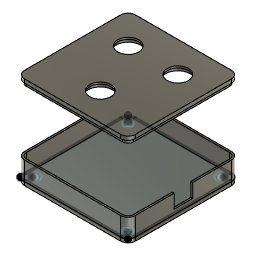
Synthetic_SCG_Actuator_Housing (Autodesk Fusion 360 design; units mm, degrees)
Autodesk Fusion 360 part; units mm, degrees
note: some values were not read from the file. Set by a fixed rule: which sketch regions a step uses.
sketch "Sketch1" plane through (0, 0, 0) normal (0, 0, 1) x (1, 0, 0)
  line L0 (3, 0) -> (55, 0)
  line L1 (58, 3) -> (58, 55)
  line L2 (55, 58) -> (3, 58)
  line L3 (0, 55) -> (0, 3)
  circle A0 centre (4, 54) radius 2.25
  circle A1 centre (54, 54) radius 2.25
  circle A2 centre (54, 4) radius 2.25
  circle A3 centre (4, 4) radius 2.25
  arc A4 (3, 58) -> (0, 55) centre (3, 55) ccw
  arc A5 (58, 55) -> (55, 58) centre (55, 55) ccw
  arc A6 (55, 0) -> (58, 3) centre (55, 3) ccw
  arc A7 (0, 3) -> (3, 0) centre (3, 3) ccw
  line L4 (55, 59) -> (3, 59)
  arc A8 (3, 59) -> (-1, 55) centre (3, 55) ccw
  line L5 (-1, 55) -> (-1, 3)
  arc A9 (-1, 3) -> (3, -1) centre (3, 3) ccw
  line L6 (3, -1) -> (55, -1)
  arc A10 (55, -1) -> (59, 3) centre (55, 3) ccw
  line L7 (59, 3) -> (59, 55)
  arc A11 (59, 55) -> (55, 59) centre (55, 55) ccw
  point P0 (58, 0)
  point P1 (0, 58)
  dimension "d1" = 58
  dimension "d2" = 58
  dimension "d5" = 4.5
  dimension "d12" = 4.5
  dimension "d13" = 4.5
  dimension "d14" = 4.5
  dimension "d15" = 3
  dimension "d16" = 3
  dimension "d17" = 3
  dimension "d18" = 3
  dimension "d19" = 1
  constraint horizontal L0
  constraint vertical L1
  constraint horizontal L2
  constraint vertical L3
  constraint coincident P1 L2
  constraint coincident P1 L3
  constraint tangent L2 A4
  constraint tangent L3 A4
  constraint tangent L2 A5
  constraint tangent L1 A5
  constraint coincident P0 L1
  constraint coincident P0 L0
  constraint tangent L1 A6
  constraint tangent L0 A6
  constraint coincident origin L0
  constraint coincident origin L3
  constraint tangent L0 A7
  constraint tangent L3 A7
  measures "d1" distance of origin P0
  measures "d2" distance of origin P1
  measures "d5" diameter of A0
  measures "d12" diameter of A1
  measures "d13" diameter of A2
  measures "d14" diameter of A3
  measures "d15" radius of A4
  measures "d16" radius of A5
  measures "d17" radius of A6
  measures "d18" radius of A7
extrude "Extrude1" add sketch "Sketch1" along normal blind 10 contours L4 A8 L5 A9 L6 A10 L7 A11 makes body 1
ref_plane "WorkPlane1" through (29, 29, 46) normal (0, 0, 1) x (1, 0, 0)
sketch "Sketch2" plane through (29, 29, 46) normal (0, 0, 1) x (1, 0, 0)
  line L0 (26, -29) -> (-26, -29)
  arc A0 (-29, -26) -> (-26, -29) centre (-26, -26) ccw
  line L1 (-29, -26) -> (-29, 26)
  arc A1 (-30, -26) -> (-26, -30) centre (-26, -26) ccw
  line L2 (-26, -30) -> (26, -30)
  arc A2 (26, -30) -> (30, -26) centre (26, -26) ccw
  arc A3 (26, -29) -> (29, -26) centre (26, -26) ccw
  line L3 (29, 26) -> (29, -26)
  line L4 (30, -26) -> (30, 26)
  arc A4 (30, 26) -> (26, 30) centre (26, 26) ccw
  arc A5 (29, 26) -> (26, 29) centre (26, 26) ccw
  line L5 (-26, 29) -> (26, 29)
  line L6 (26, 30) -> (-26, 30)
  line L7 (-30, 26) -> (-30, -26)
  arc A6 (-26, 29) -> (-29, 26) centre (-26, 26) ccw
  arc A7 (-26, 30) -> (-30, 26) centre (-26, 26) ccw
  arc A8 (-26, 27.5) -> (-27.5, 26) centre (-26, 26) ccw
  line L8 (-27.5, -26) -> (-27.5, 26)
  arc A9 (-27.5, -26) -> (-26, -27.5) centre (-26, -26) ccw
  line L9 (26, -27.5) -> (-26, -27.5)
  arc A10 (26, -27.5) -> (27.5, -26) centre (26, -26) ccw
  line L10 (27.5, 26) -> (27.5, -26)
  arc A11 (27.5, 26) -> (26, 27.5) centre (26, 26) ccw
  line L11 (-26, 27.5) -> (26, 27.5)
  dimension "d25" = 1.5
extrude "Extrude3" add sketch "Sketch2" along normal blind 2 separate body contours L0 A0 L1 A3 L3 A5 L5 A6 | A1 L2 A2 L4 A4 L6 L7 A7 | A8 L8 A9 L9 A10 L10 A11 L11 makes body 2
sketch "Sketch3" plane through (0, 0, 48) normal (0, 0, 1) x (-1, 0, 0)
  arc A0 (-3, -59) -> (1, -55) centre (-3, -55) ccw
  line L0 (1, -55) -> (1, -3)
  arc A1 (1, -3) -> (-3, 1) centre (-3, -3) ccw
  line L1 (-3, 1) -> (-55, 1)
  arc A2 (-55, 1) -> (-59, -3) centre (-55, -3) ccw
  line L2 (-59, -3) -> (-59, -55)
  arc A3 (-59, -55) -> (-55, -59) centre (-55, -55) ccw
  line L3 (-55, -59) -> (-3, -59)
  line L4 (-29, 1) -> (-29, -59)
  line L5 (-15.6061, -59) -> (-15.6061, -42.5464)
  line L6 (-39, -24.0099) -> (-19, -24.0099)
  line L7 (-19, -24.0099) -> (-19, -4.0099)
  line L8 (-19, -4.0099) -> (-39, -4.0099)
  line L9 (-39, -4.0099) -> (-39, -24.0099)
  line L10 (-39, -24.0099) -> (-19, -4.0099) construction
  line L11 (-19, -24.0099) -> (-39, -4.0099) construction
  line L12 (-25.6061, -32.5464) -> (-5.6061, -32.5464)
  line L13 (-5.6061, -32.5464) -> (-5.6061, -52.5464)
  line L14 (-5.6061, -52.5464) -> (-25.6061, -52.5464)
  line L15 (-25.6061, -52.5464) -> (-25.6061, -32.5464)
  line L16 (-25.6061, -32.5464) -> (-5.6061, -52.5464) construction
  line L17 (-5.6061, -32.5464) -> (-25.6061, -52.5464) construction
  line L18 (-32.3939, -52.5464) -> (-32.3939, -32.5464)
  line L19 (-52.3939, -52.5464) -> (-32.3939, -52.5464)
  line L20 (-52.3939, -32.5464) -> (-52.3939, -52.5464)
  line L21 (-32.3939, -32.5464) -> (-52.3939, -32.5464)
  line L22 (-52.3939, -32.5464) -> (-32.3939, -52.5464) construction
  line L23 (-32.3939, -32.5464) -> (-52.3939, -52.5464) construction
  circle A4 centre (-15.6061, -42.5464) radius 5.7
  circle A5 centre (-42.3939, -42.5464) radius 5.7
  circle A6 centre (-29, -14.0099) radius 5.7
  point P0 (-29, -14.0099)
  point P1 (-29, -14.0099)
  point P2 (-15.6061, -42.5464)
  point P3 (-42.3939, -42.5464)
  dimension "d32" = 20
  dimension "d33" = 20
  dimension "d34" = 20
  dimension "d35" = 20
  dimension "d67" = 11.4
  dimension "d68" = 11.4
  dimension "d69" = 11.4
  constraint midpoint L1 L4.start
  constraint midpoint L3 L4.end
  constraint coincident L3 L5.start
  constraint perpendicular L3 L5
  constraint horizontal L6
  constraint perpendicular L6 L7
  constraint parallel L6 L8
  constraint parallel L7 L9
  constraint coincident L10 P1
  constraint coincident L11 P1
  constraint coincident L4 P1
  constraint horizontal L12
  constraint perpendicular L12 L13
  constraint parallel L12 L14
  constraint parallel L13 L15
  constraint coincident L16 P2
  constraint coincident L17 P2
  constraint coincident P2 L5.end
  constraint symmetric L4 L12.start L18.end
  constraint symmetric L4 L12.end L20.start
  constraint symmetric L4 L13.end L19.start
  constraint symmetric L4 L14.end L18.start
  constraint symmetric L4 P2 P3
  constraint coincident P3 A5.centre
  constraint coincident P1 P0
  measures "d32" distance of L7.end L8.end
  measures "d33" distance of L6.end L7.end
  measures "d34" distance of L13.end L14.end
  measures "d35" distance of L12.end L13.end
  measures "d67" diameter of A4
  measures "d68" diameter of A5
  measures "d69" diameter of A6
extrude "Extrude9" add sketch "Sketch2" against normal blind 1 contours A8 L8 A9 L9 A10 L10 A11 L11 bodies 2
extrude "Extrude11" cut sketch "Sketch3" against normal blind 32 contours L4 A6 | L4 A6 | A4 | A5 bodies 2
sketch "Sketch5" plane through (59, 0, 0) normal (1, 0, 0) x (0, 1, 0)
  line L0 (3, 0) -> (55, 0)
  line L1 (55, 0) -> (55, 10)
  line L2 (55, 10) -> (3, 10)
  line L3 (3, 10) -> (3, 0)
  line L4 (34, 2.5) -> (24, 2.5)
  line L5 (24, 2.5) -> (24, 10.5)
  line L6 (24, 10.5) -> (34, 10.5)
  line L7 (34, 10.5) -> (34, 2.5)
  line L8 (34, 2.5) -> (24, 10.5) construction
  line L9 (24, 2.5) -> (34, 10.5) construction
  point P0 (29, 6.5)
  dimension "d47" = 10
  dimension "d48" = 8
  constraint horizontal L4
  constraint perpendicular L4 L5
  constraint parallel L4 L6
  constraint parallel L5 L7
  constraint coincident L8 P0
  constraint coincident L9 P0
  measures "d47" distance of L5.end L6.end
  measures "d48" distance of L4.end L5.end
extrude "Extrude6" cut sketch "Sketch5" against normal blind 6 contours L2 L5 L6 L7 | L2 L4 L5 L7 bodies 1
extrude "Extrude7" add sketch "Sketch2" against normal blind 2 contours L0 A0 L1 A3 L3 A5 L5 A6 bodies 2
extrude "Extrude8" add sketch "Sketch1" against normal blind 2 contours L0 L1 L2 L3 A4 A5 A6 A7 | L4 A8 L5 A9 L6 A10 L7 A11 bodies 1
sketch "Sketch7" plane through (0, 0, 45) normal (0, 0, -1) x (1, 0, 0)
  circle A0 centre (15.6061, -42.5464) radius 5.7
  circle A1 centre (42.3939, -42.5464) radius 5.7
  circle A2 centre (29, -14.0099) radius 5.7
  arc A3 (3, -1.5) -> (1.5, -3) centre (3, -3) ccw
  line L0 (1.5, -3) -> (1.5, -55)
  arc A4 (1.5, -55) -> (3, -56.5) centre (3, -55) ccw
  line L1 (3, -56.5) -> (55, -56.5)
  arc A5 (55, -56.5) -> (56.5, -55) centre (55, -55) ccw
  line L2 (56.5, -55) -> (56.5, -3)
  arc A6 (56.5, -3) -> (55, -1.5) centre (55, -3) ccw
  line L3 (55, -1.5) -> (3, -1.5)
  circle A7 centre (29, -14.0099) radius 6.7
  circle A8 centre (15.6061, -42.5464) radius 6.7
  circle A9 centre (42.3939, -42.5464) radius 6.7
  dimension "d72" = 13.4
  dimension "d73" = 13.4
  dimension "d74" = 13.4
  constraint concentric A2 A7
  constraint concentric A0 A8
  constraint concentric A1 A9
  measures "d72" diameter of A7
  measures "d73" diameter of A8
  measures "d74" diameter of A9
extrude "Extrude12" cut sketch "Sketch7" against normal blind 2 contours A7 | A8 | A9 bodies 2
